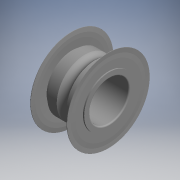
# Autodesk Inventor part: W 638/3-2Z_PART1
Saved by Autodesk Inventor 2017.3 (Build 213256000, 256)
## iProperties
Part Number: W 638/3-2Z_PART1
Material: Generic
Catalog Web Link: www.cadenas.de
Description: -Deep groove ball bearings
Vendor: SKF
Document SubType Name: Modeling
Designer: partserver
Manufacturer: SKF
Mass: 0.0217129 g
Surface Area: 1.61431 cm^2
Volume: 0.0217129 cm^3
Density: 1 g/cm^3
Appearance: PSOLRGB-175-175-175
Category: PARTsolutions
Company: SKF
Title: W 638/3-2Z_PART1
Author: Cadenas PARTsolutions
Comments: Deep groove ball bearings
PSOL_IDENT_0: {$CADENAS_DATA\23d-libs\skf_r32\bearings_units_and_housings\ball_bearings\deep_groove_ball_bearings\
PSOL_IDENT_1: bb1_001_101.prj},199 {VTYP=3D},{NB=W 638/3-2Z_PART1},{LINA=W 638/3-2Z_PART1},{NN=BB1_001_101_PART1},
PSOL_IDENT_2: {NOPRJ=TRUE},{DATE=03.04.2020 14:22:31},{GEOMDATE=30.03.2020 16:10:03},{VERSION=},{LINEID=19220},{WB
PSOL_IDENT_3: VAR=},{WBNUMERIC=}  {NB=W 638/3-2Z_PART1},{LINA=W 638/3-2Z_PART1},{KT=DUMMY},{DESIGNATION=W 638/3-2Z
PSOL_IDENT_4: },{DD=3.000},{D=7.000},{B=3.000},{C=0.000},{DD1=0.00},{DD2=3.90},{D1=0.00},{D2=6.35},{D3=0.000},{D4=
PSOL_IDENT_5: 0.000},{HH=MIN},{BB=0.000},{FF=0.00},{R0MAX=MIN},{R0=MIN},{R12=0.10},{PITCH=5.00},{DW=1.000},{DDAMIN=
PSOL_IDENT_6: 3.700},{DDAMAX=3.800},{DDBMIN=MIN},{DDBMAX=MIN},{DBMIN=MIN},{DAMAX=6.500},{BBAMIN=MIN},{CAMAX=MIN},{
PSOL_IDENT_7: RAMAX=0.100},{LOAD1=0.178},{LOAD2=0.057},{LOAD3=0.002},{SPEED1=160000},{SPEED2=80000},{KR=0.020},{F0=
PSOL_IDENT_8: 7.100},{Z=8},{II=1},{MASS=0.000},{BEARING=W 638/3-2Z},{RING=},{HELP=0.665},{HELP2=0.325},{DD1ALG=2.0
PSOL_IDENT_9: 00},{YALG=2.175},{PITCH1=5.000},{DW1=1.000},{YALG1=2.835},{HALG1=0.665},{SH=1.950},{CU=0.400},{DESIG
PSOL_IDENT_10: N=dgbbw2z},{HALG=0.675},{B1=0},{SHIELDHELP=2}
NB: W 638/3-2Z_PART1
NT: Deep groove ball bearings
NBSYN: $DESIGNATION._PART1
LINA: W 638/3-2Z_PART1
CATALOG: SKF
SUPPLIER: SKF
ARTICLENO: W 638/3-2Z_PART1
BOMINFO: W 638/3-2Z_PART1
CREATOR: CADENAS GmbH
Autodesk Inventor part; units mm, degrees
ref_plane "YZ Plane" through (0, 0, 0) normal (1, 0, 0) x (0, 1, 0)
ref_plane "XZ Plane" through (0, 0, 0) normal (0, 1, 0) x (-1, 0, 0)
ref_plane "XY Plane" through (0, 0, 0) normal (0, 0, 1) x (1, 0, 0)
sketch "Sketch_18" plane through (0, 0, 0) normal (0, 0, 1) x (1, 0, 0)
  line L0 (50, 0) -> (-50, 0)
  arc A0 (0, 1.6) -> (0.1, 1.5) centre (0.1, 1.6) ccw
  line L1 (0.1, 1.5) -> (2.9, 1.5)
  arc A1 (2.9, 1.5) -> (3, 1.6) centre (2.9, 1.6) ccw
  line L2 (3, 1.6) -> (3, 2.175)
  line L3 (3, 2.175) -> (1.88, 2.175)
  arc A2 (1.12, 2.175) -> (1.88, 2.175) centre (1.5, 2.5) ccw
  line L4 (1.12, 2.175) -> (0, 2.175)
  line L5 (0, 2.175) -> (0, 1.6)
  constraints: 12 end point, 6 point on circle, 3 centre point
revolve "Revolution1" add sketch "Sketch_18" angle 360 about axis through (50, 0, 0) along (1, 0, 0)
sketch "Sketch_19" plane through (0, 0, 0) normal (0, 0, 1) x (1, 0, 0)
  line L0 (50, 0) -> (-50, 0)
  line L1 (0, 2.575) -> (0, 1.95)
  line L2 (0, 1.95) -> (0.2333, 1.95)
  arc A0 (0.2333, 1.95) -> (0.4, 2.1167) centre (0.2333, 2.1167) ccw
  line L3 (0.4, 2.1167) -> (0.4, 2.3083)
  line L4 (0.4, 2.3083) -> (2.6, 2.3083)
  line L5 (2.6, 2.3083) -> (2.6, 2.1167)
  arc A1 (2.6, 2.1167) -> (2.7667, 1.95) centre (2.7667, 2.1167) ccw
  line L6 (2.7667, 1.95) -> (3, 1.95)
  line L7 (3, 1.95) -> (3, 2.575)
  line L8 (3, 2.575) -> (0, 2.575)
  constraints: 18 end point, 4 point on circle, 2 centre point
revolve "Revolution2" cut sketch "Sketch_19" angle 360 about axis through (50, 0, 0) along (1, 0, 0)
sketch "Sketch_20" plane through (0, 0, 0) normal (0, 0, 1) x (1, 0, 0)
  line L0 (50, 0) -> (-50, 0)
  line L1 (0.09, 3.175) -> (0.105, 2.8662)
  line L2 (0.105, 2.8662) -> (0.09, 2.5575)
  line L3 (0.09, 2.5575) -> (0.09, 1.94)
  line L4 (0.09, 1.94) -> (0.12, 1.94)
  line L5 (0.12, 1.94) -> (0.15, 2.5575)
  line L6 (0.15, 2.5575) -> (0.15, 2.8662)
  line L7 (0.15, 2.8662) -> (0.12, 3.175)
  line L8 (0.12, 3.175) -> (0.09, 3.175)
  constraints: 18 end point
revolve "Revolution3" add sketch "Sketch_20" angle 360 about axis through (50, 0, 0) along (1, 0, 0)
sketch "Sketch_21" plane through (0, 0, 0) normal (0, 0, 1) x (1, 0, 0)
  line L0 (50, 0) -> (-50, 0)
  line L1 (2.85, 2.8662) -> (2.85, 2.5575)
  line L2 (2.85, 2.5575) -> (2.88, 1.94)
  line L3 (2.88, 1.94) -> (2.91, 1.94)
  line L4 (2.91, 1.94) -> (2.91, 2.5575)
  line L5 (2.91, 2.5575) -> (2.895, 2.8662)
  line L6 (2.895, 2.8662) -> (2.91, 3.175)
  line L7 (2.91, 3.175) -> (2.88, 3.175)
  line L8 (2.88, 3.175) -> (2.85, 2.8662)
  constraints: 18 end point
revolve "Revolution4" add sketch "Sketch_21" angle 360 about axis through (50, 0, 0) along (1, 0, 0)
body "Solid1"
